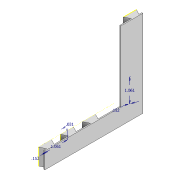
# Autodesk Inventor part: Sliding test wall
Saved by Autodesk Inventor 2020 (Build 240168000, 168)
## iProperties
Created: 2019-11-10
Part Number: Sliding test wall
Material: Generic
Document SubType Name: Modeling
Designer: ball
Density: 1 g/cm^3
Appearance: Default
Author: ball
Autodesk Inventor part; units mm, degrees
ref_plane "YZ Plane" through (0, 0, 0) normal (1, 0, 0) x (0, 1, 0)
ref_plane "XZ Plane" through (0, 0, 0) normal (0, 1, 0) x (-1, 0, 0)
ref_plane "XY Plane" through (0, 0, 0) normal (0, 0, 1) x (1, 0, 0)
sketch "Sketch1" plane through (0, 0, 0) normal (0, 1, 0) x (-1, 0, 0)
  line L0 (0, 4.5) -> (0.254, 4.5)
  line L1 (0.254, -4.5) -> (0, -4.5)
  line L2 (6.35, 4.5) -> (6.35, -4.5)
  line L3 (6.35, 7.548) -> (6.35, 4.5)
  line L4 (6.35, -7.548) -> (6.35, -4.5)
  line L5 (0.254, 4.5) -> (6.35, 7.548)
  line L6 (0.254, -4.5) -> (6.35, -7.548)
  line L7 (0, 4.5) -> (0, -4.5)
  line L8 (0, -20.9) -> (0.254, -20.9)
  line L9 (0.254, -29.9) -> (0, -29.9)
  line L10 (6.35, -20.9) -> (6.35, -29.9)
  line L11 (6.35, -17.852) -> (6.35, -20.9)
  line L12 (6.35, -32.948) -> (6.35, -29.9)
  line L13 (0.254, -20.9) -> (6.35, -17.852)
  line L14 (0.254, -29.9) -> (6.35, -32.948)
  line L15 (0, -20.9) -> (0, -29.9)
  line L16 (0, -46.3) -> (0.254, -46.3)
  line L17 (0.254, -55.3) -> (0, -55.3)
  line L18 (6.35, -46.3) -> (6.35, -55.3)
  line L19 (6.35, -43.252) -> (6.35, -46.3)
  line L20 (6.35, -58.348) -> (6.35, -55.3)
  line L21 (0.254, -46.3) -> (6.35, -43.252)
  line L22 (0.254, -55.3) -> (6.35, -58.348)
  line L23 (0, -46.3) -> (0, -55.3)
  line L24 (0, -71.7) -> (0.254, -71.7)
  line L25 (0.254, -80.7) -> (0, -80.7)
  line L26 (6.35, -71.7) -> (6.35, -80.7)
  line L27 (6.35, -68.652) -> (6.35, -71.7)
  line L28 (6.35, -83.748) -> (6.35, -80.7)
  line L29 (0.254, -71.7) -> (6.35, -68.652)
  line L30 (0.254, -80.7) -> (6.35, -83.748)
  line L31 (0, -71.7) -> (0, -80.7)
  point P0 (0, 0)
  dimension "d16" = 6.096
  dimension "d25" = 9
  dimension "d26" = 3.048
  dimension "d27" = 3.048
  dimension "d28" = 0.254
  dimension "d29" = 0.254
  dimension "d33" = 25.4
  constraints: 64 end point, 4 point on line, 2 vertical, 1 collinear, 1 horizontal, 1 parallel, 53 other
  measures "d16" distance from line of L4 L1.start
  measures "d25" distance between parallel lines of L0 L1
  measures "d26" vertical distance of L0.end L3.start
  measures "d27" vertical distance of L4.start L1.start
  measures "d28" distance of L1.end L1.start
  measures "d29" distance of L0.start L0.end
  measures "d33" distance of L0.start L8.start
extrude "Shape" add sketch "Sketch1" along normal blind 19.05 contours L0 L5 L3 L2 L4 L6 L1 L7 | L8 L13 L11 L10 L12 L14 L9 L15 | L16 L21 L19 L18 L20 L22 L17 L23
sketch "Sketch4" plane through (0, 0, 0) normal (0, -1, 0) x (1, 0, 0)
  line L0 (0, -55.3) -> (-0.254, -55.3) construction
  line L1 (0, -46.3) -> (0, -55.3) construction
  line L2 (-6.35, -43.252) -> (-0.254, -46.3) construction
  line L3 (-6.35, -58.348) -> (-6.35, -43.252) construction
  line L4 (-0.254, -55.3) -> (-6.35, -58.348) construction
  line L5 (-0.254, -46.3) -> (0, -46.3) construction
  line L6 (0, -93.6625) -> (-0.254, -93.6625)
  line L7 (-0.254, -93.6625) -> (-6.35, -90.6145)
  line L8 (-6.35, -105.7105) -> (-6.35, -90.6145)
  line L9 (-0.254, -55.3) -> (-6.35, -58.348) projected
  line L10 (-0.254, -102.6625) -> (-6.35, -105.7105)
  line L11 (0, -102.6625) -> (-0.254, -102.6625)
  line L12 (0, -102.6625) -> (0, -93.6625)
  line L13 (-0.254, -46.3) -> (0, -46.3) projected
  line L14 (0, -46.3) -> (0, -55.3) projected
  line L15 (0, -55.3) -> (0, -93.4) construction
  point P0 (0, 0)
  dimension "d43" = 38.1
  constraints: 14 end point, 3 vertical, 2 horizontal, 2 parallel
  measures "d43" distance of L0.start L15.end
extrude "Extrusion4" add sketch "Sketch4" against normal blind 100.2792
sketch "Sketch5" plane through (0, 0, -93.6625) normal (1, 0, 0) x (0, 0, -1)
  line L0 (12.048, 0) -> (12.048, 100.2792) construction
  line L1 (0, 100.2792) -> (9, 100.2792) construction
  line L2 (-101.2105, 0) -> (-101.2105, 19.05) construction
  line L3 (-86.1145, 0) -> (-101.2105, 0) projected
  line L4 (12.048, 0) -> (9, 0) projected
  line L5 (-101.2105, 0) -> (12.048, 0)
  line L6 (9, 100.2792) -> (12.048, 100.2792) projected
  line L7 (12.048, 0) -> (12.048, 100.2792)
  line L8 (12.048, 100.2792) -> (-13.352, 100.2792)
  line L9 (-13.352, 100.2792) -> (-13.352, 19.05)
  line L10 (-38.3625, 19.05) -> (-35.3145, 19.05) projected
  line L11 (-86.1145, 19.05) -> (-101.2105, 19.05) projected
  line L12 (-13.352, 19.05) -> (-101.2105, 19.05)
  line L13 (-101.2105, 19.05) -> (-101.2105, 0)
  point P0 (-93.6625, 0)
  point P1 (-101.2105, 100.2792)
  dimension "d46" = 25.4
  constraints: 12 end point, 4 perpendicular, 2 horizontal, 1 point on line
  measures "d46" distance of L0.end L8.end
extrude "Extrusion5" add sketch "Sketch5" along normal blind 1.27
sketch "Sketch6" plane through (-6.35, 0, -105.7105) normal (-1, 0, 0) x (0, 0, 1)
  line L0 (0, 100.2792) -> (15.096, 100.2792) projected
  line L1 (7.548, 100.2792) -> (7.548, 0) construction
  line L2 (113.2585, 0) -> (0, 0) projected
  circle A0 centre (7.548, 9.525) radius 1.9304
  circle A1 centre (7.548, 36.4744) radius 1.9304
  circle A2 centre (7.548, 63.4238) radius 1.9304
  circle A3 centre (7.548, 90.3732) radius 1.9304
  circle A4 centre (106.4852, 9.525) radius 1.9304
  circle A5 centre (79.5358, 9.525) radius 1.9304
  line L3 (113.2585, 0) -> (113.2585, 19.05) projected
  line L4 (25.4, 19.05) -> (113.2585, 19.05) construction
  line L5 (105.7105, 19.05) -> (105.7105, 0) construction
  line L6 (72.7625, 19.05) -> (87.8585, 19.05) construction
  line L7 (80.3105, 19.05) -> (80.3105, 0) construction
  line L8 (72.7625, 0) -> (87.8585, 0) construction
  line L9 (72.7625, 0) -> (72.7625, 19.05) projected
  line L10 (87.8585, 0) -> (87.8585, 19.05) projected
  dimension "d54" = 26.9494
  dimension "d48" = 3.8608
  dimension "d51" = 26.9494
  dimension "d57" = 3.8608
  dimension "d60" = 26.9494
  dimension "d69" = 0.7747
  constraints: 6 centre point, 6 end point, 3 midpoint, 3 point on line, 2 horizontal, 2 vertical, 1 perpendicular, 8 other
  measures "d48" diameter of A0
  measures "d51" distance of A0.centre A1.centre
  measures "d57" diameter of A4
  measures "d60" distance of A4.centre A5.centre
  measures "d69" distance from line of L7 A5.centre
equation "\"d27\" = d26"
equation "\"d29\" = d28"
body "Solid1"
